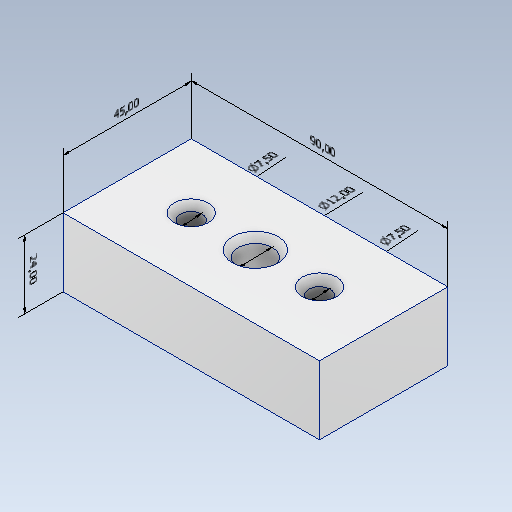
# Autodesk Inventor part: sujecion_castor
Saved by Autodesk Inventor 2021 (Build 250183000, 183)
## iProperties
Created: 2020-10-29
Part Number: sujecion_castor
Material: Aluminio 6061
Document SubType Name: Modeling
Designer: germi
Density: 2.7 g/cm^3
Appearance: Aluminio - Plano
Mass: 196.755 g
Surface Area: 143.488 cm^2
Volume: 72.8721 cm^3
Author: germi
Autodesk Inventor part; units mm, degrees
ref_plane "YZ Plane" through (0, 0, 0) normal (1, 0, 0) x (0, 1, 0)
ref_plane "XZ Plane" through (0, 0, 0) normal (0, 1, 0) x (-1, 0, 0)
ref_plane "XY Plane" through (0, 0, 0) normal (0, 0, 1) x (1, 0, 0)
sketch "Boceto1" plane through (0, 0, 0) normal (0, 1, 0) x (-1, 0, 0)
  line L0 (45, 22.5) -> (-45, 22.5)
  line L1 (-45, 22.5) -> (-45, -22.5)
  line L2 (-45, -22.5) -> (45, -22.5)
  line L3 (45, -22.5) -> (45, 22.5)
  point P0 (-45, 0)
  constraints: 8 end point, 2 parallel, 1 horizontal, 1 perpendicular
extrude "Extrusión1" add sketch "Boceto1" along normal blind 24
sketch "Boceto2" plane through (0, 24, 0) normal (0, 1, 0) x (1, 0, 0)
  point P0 (-22.5, 0)
hole "Agujero1" at (-22.5, 24, 0) direction (0, -1, 0) diameter 7.5 end through all countersink diameter 12 countersink angle 90
sketch "Boceto3" plane through (0, 24, 0) normal (0, 1, 0) x (1, 0, 0)
  point P0 (0, 0)
hole "Agujero2" at (0, 24, 0) direction (0, -1, 0) diameter 12 end through all countersink diameter 16 countersink angle 82
sketch "Boceto4" plane through (0, 24, 0) normal (0, 1, 0) x (1, 0, 0)
  point P0 (0, 0)
  point P1 (0, 0)
  point P2 (22.5, 0)
  constraints: 1 coincident
hole "Agujero3" at (0, 24, 0) at (22.5, 24, 0) direction (0, -1, 0) diameter 7.5 end through all countersink diameter 12 countersink angle 82
